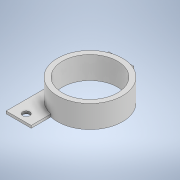
# Autodesk Inventor part: Ball_Bearing_Holder
Saved by Autodesk Inventor 2022 (Build 260153000, 153)
## iProperties
Created: 2023-03-18
Part Number: Ball_Bearing_Holder
Material: Generic
Document SubType Name: Modeling
Designer: zarek
Density: 1 g/cm^3
Appearance: Default
Author: zarek
Autodesk Inventor part; units mm, degrees
ref_plane "YZ Plane" through (0, 0, 0) normal (1, 0, 0) x (0, 1, 0)
ref_plane "XZ Plane" through (0, 0, 0) normal (0, 1, 0) x (-1, 0, 0)
ref_plane "XY Plane" through (0, 0, 0) normal (0, 0, 1) x (1, 0, 0)
sketch "Sketch3" plane through (0, 0, 0) normal (0, 1, 0) x (-1, 0, 0)
  line L0 (3, -20.5) -> (3, -14.5)
  line L1 (13, 20.5) -> (3, 20.5)
  line L2 (3, -20.5) -> (3, 20.5)
  line L3 (3, 20.5) -> (13, 20.5)
  line L4 (13, 20.5) -> (13, -20.5)
  line L5 (13, -20.5) -> (3, -20.5)
  line L6 (0, 0) -> (3, 0)
  line L7 (13, 14.5) -> (3, 14.5)
  line L8 (3, -14.5) -> (13, -14.5)
  line L9 (3, -14.5) -> (13, -14.5)
  line L10 (3, 14.5) -> (13, 14.5)
  circle A0 centre (8, -17.508) radius 1.425
  circle A1 centre (8, -17.508) radius 1.425
  circle A2 centre (8, 17.4854) radius 1.425
  circle A3 centre (8, 17.4854) radius 1.425
  point P0 (3, 20.5)
  dimension "d15" = 41
  dimension "d16" = 10
  dimension "d17" = 0
  dimension "d18" = 6
  constraints: 22 end point, 4 centre point, 4 equal length, 2 coincident, 1 midpoint, 1 perpendicular
  measures "d15" distance of L1.start L4.end
  measures "d16" distance between parallel lines of L4 L2
  measures "d17" vertical distance of L6.start L6.end
  measures "d18" distance between parallel lines of L1 L7
extrude "Extrusion1" add sketch "Sketch3" along normal blind 1
sketch "Sketch5" plane through (0, 0, 0) normal (0, -1, 0) x (1, 0, 0)
  line L0 (-3, 20.5) -> (-3, 14.5)
  line L1 (-13, -20.5) -> (-3, -20.5)
  line L2 (-3, 20.5) -> (-3, -20.5)
  line L3 (-3, -20.5) -> (-13, -20.5)
  line L4 (-13, -20.5) -> (-13, 20.5)
  line L5 (-13, 20.5) -> (-3, 20.5)
  line L6 (0, 0) -> (-3, 0)
  line L7 (-13, -14.5) -> (-3, -14.5)
  line L8 (-3, 14.5) -> (-13, 14.5)
  line L9 (-3, 14.5) -> (-13, 14.5)
  line L10 (-3, -14.5) -> (-13, -14.5)
  circle A0 centre (-8, 17.508) radius 1.425
  circle A1 centre (-8, 17.508) radius 1.425
  circle A2 centre (-8, -17.4854) radius 1.425
  circle A3 centre (-8, -17.4854) radius 1.425
  circle A4 centre (0, 0) radius 11
  circle A5 centre (0, 0) radius 13
  point P0 (3, 20.5)
  point P1 (3, -14.5)
  point P2 (-3, 12.6491)
  point P3 (-3, 10.583)
  point P4 (-3, -10.583)
  point P5 (-3, -12.6491)
  dimension "d27" = 41
  dimension "d28" = 10
  dimension "d29" = 0
  dimension "d30" = 6
  dimension "d31" = 22
  dimension "d32" = 26
  constraints: 22 end point, 6 centre point, 4 coincident, 4 equal length, 1 midpoint, 1 perpendicular
  measures "d27" distance of L1.start L4.end
  measures "d28" distance between parallel lines of L4 L2
  measures "d29" vertical distance of L6.start L6.end
  measures "d30" distance between parallel lines of L1 L7
  measures "d31" diameter of A4
  measures "d32" diameter of A5
extrude "Extrusion2" add sketch "Sketch5" against normal blind 9 contours A5 L2 A4 | L2 A4 A5
sketch "Sketch6" plane through (0, 9, 0) normal (0, 1, 0) x (1, 0, 0)
  circle A0 centre (0, 0) radius 11
  constraints: 1 centre point, 1 coincident
extrude "Extrusion3" cut sketch "Sketch6" against normal through all
body "Solid1"
